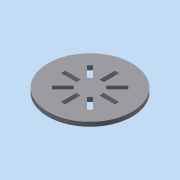
# Autodesk Inventor part: medio
Saved by Autodesk Inventor 2015 (Build 190159000, 159)
## iProperties
Created: 2017-10-02
Part Number: medio
Material: Generic
Document SubType Name: Modeling
Designer: macbook
Density: 1 g/cm^3
Appearance: Default
Author: macbook
Autodesk Inventor part; units mm, degrees
ref_plane "YZ Plane" through (0, 0, 0) normal (1, 0, 0) x (0, 1, 0)
ref_plane "XZ Plane" through (0, 0, 0) normal (0, 1, 0) x (-1, 0, 0)
ref_plane "XY Plane" through (0, 0, 0) normal (0, 0, 1) x (1, 0, 0)
sketch "Sketch1" plane through (0, 0, 0) normal (0, 0, 1) x (1, 0, 0)
  circle A0 centre (0, 0) radius 54.5
  line L0 (15, 2.8) -> (35, 2.8)
  line L1 (35, 2.8) -> (35, -2.7)
  line L2 (35, -2.7) -> (15, -2.7)
  line L3 (15, -2.7) -> (15, 2.8)
  line L4 (8.6974, 12.6158) -> (22.8395, 26.7579)
  line L5 (22.8395, 26.7579) -> (26.7286, 22.8688)
  line L6 (26.7286, 22.8688) -> (12.5865, 8.7267)
  line L7 (12.5865, 8.7267) -> (8.6974, 12.6158)
  line L8 (-2.7, 15.1) -> (-2.7, 35.1)
  line L9 (-2.7, 35.1) -> (2.8, 35.1)
  line L10 (2.8, 35.1) -> (2.8, 15.1)
  line L11 (2.8, 15.1) -> (-2.7, 15.1)
  line L12 (-12.5158, 8.7974) -> (-26.6579, 22.9395)
  line L13 (-26.6579, 22.9395) -> (-22.7688, 26.8286)
  line L14 (-22.7688, 26.8286) -> (-8.6267, 12.6865)
  line L15 (-8.6267, 12.6865) -> (-12.5158, 8.7974)
  line L16 (-15, -2.6) -> (-35, -2.6)
  line L17 (-35, -2.6) -> (-35, 2.9)
  line L18 (-35, 2.9) -> (-15, 2.9)
  line L19 (-15, 2.9) -> (-15, -2.6)
  line L20 (-8.6974, -12.4158) -> (-22.8395, -26.5579)
  line L21 (-22.8395, -26.5579) -> (-26.7286, -22.6688)
  line L22 (-26.7286, -22.6688) -> (-12.5865, -8.5267)
  line L23 (-12.5865, -8.5267) -> (-8.6974, -12.4158)
  line L24 (2.7, -14.9) -> (2.7, -34.9)
  line L25 (2.7, -34.9) -> (-2.8, -34.9)
  line L26 (-2.8, -34.9) -> (-2.8, -14.9)
  line L27 (-2.8, -14.9) -> (2.7, -14.9)
  line L28 (12.5158, -8.5974) -> (26.6579, -22.7395)
  line L29 (26.6579, -22.7395) -> (22.7688, -26.6286)
  line L30 (22.7688, -26.6286) -> (8.6267, -12.4865)
  line L31 (8.6267, -12.4865) -> (12.5158, -8.5974)
  line L32 (24.2998, 0.05) -> (27.4417, 0.05)
  point P0 (0, 0.1)
  dimension "d0" = 109
  dimension "d3" = 20
  dimension "d4" = 5.5
  dimension "d5" = 360
  dimension "d8" = 2.75
  constraints: 66 end point, 2 horizontal, 2 parallel, 1 centre point, 1 coincident, 1 perpendicular, 65 other
  measures "d0" diameter of A0
  measures "d3" distance of L1.end L3.start
  measures "d4" distance of L0.end L1.end
  measures "d8" distance between parallel lines of L0 L32
extrude "Extrusion1" add sketch "Sketch1" along normal blind 5.5
body "Solid1"
